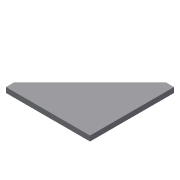
# Autodesk Inventor part: gusset
Saved by Autodesk Inventor 2022 (Build 260148000, 148)
## iProperties
Created: 2008-03-11
Part Number: gusset
Document SubType Name: Modeling
Designer: jmacmillan
Density: 1 g/cm^3
Material: Generic
Appearance: Default
Author: jmacmillan
Autodesk Inventor part; units mm, degrees
ref_plane "YZ Plane" through (0, 0, 0) normal (1, 0, 0) x (0, 1, 0)
ref_plane "XZ Plane" through (0, 0, 0) normal (0, 1, 0) x (-1, 0, 0)
ref_plane "XY Plane" through (0, 0, 0) normal (0, 0, 1) x (1, 0, 0)
sketch "Sketch1" plane through (0, 0, 0) normal (0, 0, 1) x (1, 0, 0)
  line L0 (39.1526, 75.1474) -> (39.1526, -26.4526) projected
  line L1 (-5.5514, 24.3474) -> (39.1526, 24.3474) projected
  line L2 (39.1526, 65.117) -> (35.1526, 65.117)
  line L3 (35.1526, 65.117) -> (-1.617, 28.3474)
  line L4 (-1.617, 28.3474) -> (-1.617, 24.3474)
  dimension "d0" = 4
  dimension "d1" = 4
  dimension "d2" = 45
  dimension "d3" = 52
  constraints: 6 end point, 2 point on line, 1 parallel, 1 perpendicular
  measures "d0" distance of L2.start L2.end
  measures "d1" distance of L3.end L4.end
  measures "d2" angle of L3 L0
  measures "d3" distance of L2.end L3.end
extrude "Extrusion1" add sketch "Sketch1" along normal mid plane 2.5
body "Solid1"
